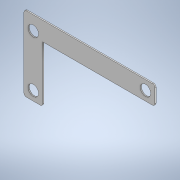
# Autodesk Inventor part: Arm
Saved by Autodesk Inventor 2020 (Build 240168000, 168)
## iProperties
Created: 2020-01-26
Part Number: Arm
Material: Generic
Document SubType Name: Modeling
Designer: autum
Density: 1 g/cm^3
Appearance: Default
Author: autum
Autodesk Inventor part; units mm, degrees
ref_plane "YZ Plane" through (0, 0, 0) normal (1, 0, 0) x (0, 1, 0)
ref_plane "XZ Plane" through (0, 0, 0) normal (0, 1, 0) x (-1, 0, 0)
ref_plane "XY Plane" through (0, 0, 0) normal (0, 0, 1) x (1, 0, 0)
sketch "Sketch1" plane through (0, 0, 0) normal (0, 0, 1) x (1, 0, 0)
  line L0 (0, 0) -> (50.8, 0)
  line L1 (50.8, 0) -> (50.8, 152.4)
  line L2 (50.8, 203.2) -> (0, 203.2)
  line L3 (0, 203.2) -> (0, 0)
  line L4 (0, 203.2) -> (355.6, 203.2)
  line L5 (355.6, 203.2) -> (355.6, 152.4)
  line L6 (355.6, 152.4) -> (50.8, 152.4)
  line L7 (0, 152.4) -> (0, 203.2)
  dimension "d0" = 50.8
  dimension "d1" = 203.2
  dimension "d2" = 355.6
  dimension "d3" = 50.8
  constraints: 16 end point, 4 parallel, 2 horizontal, 2 perpendicular
  measures "d0" distance of L2.end L2.start
  measures "d1" distance of L2.start L0.end
  measures "d2" distance of L5.end L7.start
  measures "d3" distance of L4.end L5.end
extrude "Extrusion1" add sketch "Sketch1" along normal blind 3.175
sketch "Sketch2" plane through (0, 0, 3.175) normal (0, 0, 1) x (1, 0, 0)
  line L0 (355.6, 203.2) -> (0, 203.2) projected
  line L1 (0, 203.2) -> (0, 0) projected
  point P0 (25.4, 165.1)
  dimension "d20" = 38.1
  dimension "d21" = 25.4
  measures "d20" distance from line of L0 point (25.4, 165.1)
  measures "d21" distance from line of L1 point (25.4, 165.1)
hole "Hole1" at (25.4, 165.1, 3.175) direction (0, 0, -1) diameter 28.575 end through all
sketch "Sketch3" plane through (0, 0, 3.175) normal (0, 0, 1) x (1, 0, 0)
  line L0 (50.8, 0) -> (50.8, 152.4) projected
  line L1 (0, 0) -> (50.8, 0) projected
  point P0 (25.4, 25.4)
  dimension "d22" = 25.4
  dimension "d23" = 25.4
  measures "d22" distance from line of L0 point (25.4, 25.4)
  measures "d23" distance from line of L1 point (25.4, 25.4)
hole "Hole2" at (25.4, 25.4, 3.175) direction (0, 0, -1) diameter 28.575 end through all
fillet "Fillet1" radius 6.35 5 edges at (355.6, 152.4, 1.5875) (355.6, 203.2, 1.5875) (50.8, 0, 1.5875) (0, 0, 1.5875) (0, 203.2, 1.5875)
sketch "Sketch4" plane through (0, 0, 3.175) normal (0, 0, 1) x (1, 0, 0)
  line L0 (349.25, 203.2) -> (6.35, 203.2) projected
  line L1 (355.6, 158.75) -> (355.6, 196.85) projected
  point P0 (0, 0)
  point P1 (330.2, 177.8)
  dimension "d32" = 25.4
  dimension "d33" = 25.4
  measures "d32" distance from line of L0 point (330.2, 177.8)
  measures "d33" distance from line of L1 point (330.2, 177.8)
hole "Hole3" at (330.2, 177.8, 3.175) direction (0, 0, -1) diameter 28.575 end through all
body "Solid1"
